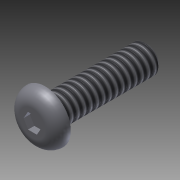
# Autodesk Inventor part: 6 32 bolt 0.5''
Saved by Autodesk Inventor 2012 (Build 160160000, 160)
## iProperties
Created: 2013-08-29
Part Number: 6 32 bolt 0.5''
Material: Default
Document SubType Name: Modeling
Designer: Bryce
Density: 1 g/cm^3
Author: Bryce
Autodesk Inventor part; units mm, degrees
ref_plane "YZ Plane" through (0, 0, 0) normal (1, 0, 0) x (0, 1, 0)
ref_plane "XZ Plane" through (0, 0, 0) normal (0, 1, 0) x (-1, 0, 0)
ref_plane "XY Plane" through (0, 0, 0) normal (0, 0, 1) x (1, 0, 0)
sketch "Sketch1" plane through (0, 0, 0) normal (0, 0, 1) x (1, 0, 0)
  circle A0 centre (0, 0) radius 3.175
  circle A1 centre (0, 0) radius 1.7272
  line L0 (0.5499, 0.9525) -> (1.0999, 0)
  line L1 (1.0999, 0) -> (0.5499, -0.9525)
  line L2 (0.5499, -0.9525) -> (-0.5499, -0.9525)
  line L3 (-0.5499, -0.9525) -> (-1.0999, 0)
  line L4 (-1.0999, 0) -> (-0.5499, 0.9525)
  line L5 (-0.5499, 0.9525) -> (0.5499, 0.9525)
  dimension "d0" = 3.4544
  dimension "d1" = 6.35
  dimension "d2" = 1.905
  constraints: 12 end point, 3 coincident, 2 centre point, 1 horizontal, 13 other
  measures "d0" diameter of A1
  measures "d1" diameter of A0
  measures "d2" distance between parallel lines of L2 L5
extrude "Extrusion1" add sketch "Sketch1" against normal blind 12.7 contours A1 | L0 L1 L2 L3 L4 L5
extrude "Extrusion2" add sketch "Sketch1" along normal blind 1.5875 contours A0 | A1
extrude "Extrusion3" add sketch "Sketch1" along normal blind 0.7937 contours L0 L1 L2 L3 L4 L5
thread "Thread1" size "6-32 UNC" class "2A" standard "ANSI Unified Screw Threads" full length
chamfer "Chamfer1" distance 0.3969 angle 45 1 edges at (-1.7272, 0, -12.7)
fillet "Fillet1" radius 1.5875 1 edges at (-3.175, 0, 1.5875)
body "Solid1"
